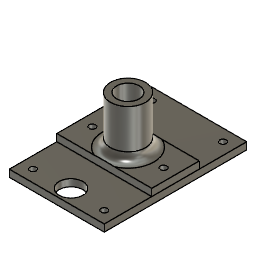
receiver_lens_15mm (Autodesk Fusion 360 design; units mm, degrees)
Autodesk Fusion 360 part; units mm, degrees
sketch "Sketch1" plane through (0, 0, 0) normal (0, 0, 1) x (1, 0, 0)
  circle A0 centre (20, 6) radius 5
  line L0 (0, 60) -> (0, 0)
  line L1 (40, 60) -> (0, 60)
  circle A1 centre (20, 30) radius 4.75
  line L2 (40, 0) -> (40, 60)
  circle A2 centre (35, 55) radius 1.35
  line L3 (0, 0) -> (40, 0)
  circle A3 centre (35, 5) radius 1.35
  circle A4 centre (20, 30) radius 6.25
  circle A5 centre (5, 5) radius 1.35
  circle A6 centre (5, 30) radius 1.35
  circle A7 centre (35, 30) radius 1.35
  circle A8 centre (5, 55) radius 1.35
  circle A9 centre (20, 30) radius 5.5
  dimension "d3" = 30
  dimension "d4" = 50
  dimension "d9" = 2.7
  dimension "d10" = 60
  dimension "d11" = 40
  dimension "d12" = 5
  dimension "d13" = 5
  dimension "d14" = 12.5
  dimension "d15" = 20
  dimension "d16" = 30
  dimension "d17" = 9.5
  dimension "d18" = 6
  dimension "d19" = 20
  dimension "d20" = 10
  dimension "d32" = 11
  constraint horizontal L3
  constraint vertical L2
  constraint horizontal L1
  constraint vertical L0
  constraint coincident L0.end L3.start
  constraint concentric A1 A4
  constraint concentric A4 A9
  measures "d9" diameter of A5
  measures "d10" distance of L2.start L1.start
  measures "d11" distance of L0.start L1.start
  measures "d12" distance of A5.centre L3
  measures "d13" distance of A5.centre L0
  measures "d14" diameter of A4
  measures "d15" distance of A1.centre L2
  measures "d16" distance of A1.centre L3
  measures "d17" diameter of A1
  measures "d18" distance of A0.centre L3
  measures "d19" distance of A0.centre L2
  measures "d20" diameter of A0
  measures "d32" diameter of A9
extrude "Extrude1" add sketch "Sketch1" along normal blind 3 contours L0 L1 L2 L3 makes body 1
extrude "Extrude2" add sketch "Sketch1" along normal blind 14 separate body contours A4 | A9 makes body 2
sketch "Sketch2" plane through (0, 0, 14) normal (0, 0, 1) x (-1, 0, 0)
  circle A0 centre (-20, -30) radius 4.75
  circle A1 centre (-20, -30) radius 6.25
  circle A2 centre (-20, -30) radius 5.5
  dimension "d33" = 11
  constraint concentric A0 A2
  measures "d33" diameter of A2
extrude "Extrude3" cut sketch "Sketch2" against normal blind 1 contours A2 bodies 2
sketch "Sketch3" plane through (0, 0, 3) normal (0, 0, 1) x (-1, 0, 0)
  circle A0 centre (-20, -30) radius 6.25
  circle A1 centre (-35, -5) radius 1.35
  circle A2 centre (-5, -55) radius 1.35
  circle A3 centre (-20, -6) radius 5
  circle A4 centre (-5, -30) radius 1.35
  circle A5 centre (-35, -30) radius 1.35
  circle A6 centre (-35, -55) radius 1.35
  circle A7 centre (-5, -5) radius 1.35
  line L0 (0, 0) -> (-40, 0)
  line L1 (-40, 0) -> (-40, -60)
  line L2 (-40, -60) -> (0, -60)
  line L3 (0, -60) -> (0, 0)
  line L4 (0, -40) -> (-40, -40)
  line L5 (-40, -40) -> (-40, -20)
  line L6 (-40, -20) -> (0, -20)
  line L7 (0, -20) -> (0, -40)
  line L8 (0, 0) -> (-40, 0)
  circle A8 centre (-20, -30) radius 6.75
  circle A9 centre (-20, -30) radius 7.35
  circle A10 centre (-35, -30) radius 1.35
  circle A11 centre (-5, -30) radius 1.35
  dimension "d36" = 20
  dimension "d37" = 20
  dimension "d38" = 14.7
  dimension "d39" = 13.5
  constraint horizontal L4
  constraint vertical L5
  constraint horizontal L6
  constraint vertical L7
  constraint coincident L1 L5.end
  constraint coincident L3 L4.start
  constraint concentric A0 A8
  constraint concentric A8 A9
  constraint concentric A5 A10
  constraint concentric A4 A11
  measures "d36" distance of L4.end L5.end
  measures "d37" distance of L6 L8
  measures "d38" diameter of A9
  measures "d39" diameter of A8
extrude "Extrude4" add sketch "Sketch3" along normal blind 3 contours L1 L3 L4 L5 L6 L7 bodies 1
extrude "Extrude5" add sketch "Sketch3" along normal blind 23 contours A9 bodies 1
sketch "Sketch4" plane through (0, 0, 26) normal (0, 0, 1) x (-1, 0, 0)
  circle A0 centre (-20, -30) radius 6.75
  circle A1 centre (-20, -30) radius 7.35
  circle A2 centre (-20, -30) radius 4.75
  dimension "d44" = 9.5
  constraint concentric A0 A2
  measures "d44" diameter of A2
extrude "Extrude6" add sketch "Sketch4" against normal blind 10.5 contours A0 bodies 1
fillet "Fillet2" radius 1.5 1 edges at (26.2932, 32.4409, 15.5) on bodies 1
split "Split1" by plane through (0, 0, 3) normal (0, 0, 1) bodies 1 makes body 3 at (12.6865, 30.7318, 19.3333)
combine "Combine1" operation add target body 2 tool bodies 1
fillet "Fillet3" radius 3.5 1 edges at (26.2932, 32.4409, 3) on bodies 3
fillet "Fillet4" radius 2 1 edges at (14.173, 27.7399, 3) on bodies 2
fillet "Fillet5" radius 3.5 1 edges at (26.8526, 27.3421, 6) on bodies 3
move_body "Move1" bodies 3 to x (1, 0, 0) y (0, 1, 0) z (0, 0, 1) at (0, 0, 10)
sketch "Sketch5" plane through (0, 0, 14) normal (0, 0, 1) x (-1, 0, 0)
  circle A0 centre (-20, -30) radius 5.5
  circle A1 centre (-20, -30) radius 6.25
  circle A2 centre (-20, -30) radius 6.25
  circle A3 centre (-20, -30) radius 5.5
  circle A4 centre (-20, -30) radius 4.75
  dimension "d59" = 12.5
  dimension "d60" = 11
  dimension "d61" = 9.5
  constraint concentric A0 A2
  constraint concentric A0 A3
  constraint concentric A0 A4
  measures "d59" diameter of A2
  measures "d60" diameter of A3
  measures "d61" diameter of A4
extrude "Extrude7" add sketch "Sketch5" along normal blind 10 separate body contours A1 A2 makes body 4
extrude "Extrude8" add sketch "Sketch5" along normal blind 9 contours A0 A3 bodies 2 4
ref_plane "WorkPlane1" through (20, 30, 14) normal (0, 0, -1) x (-1, 0, 0)
split "Split2" by plane through (20, 30, 14) normal (0, 0, -1) bodies 2 makes body 5 at (19.8817, 47.9803, 0)
sketch "Sketch6" plane through (0, 0, 3) normal (0, 0, 1) x (-1, 0, 0)
  line L0 (0, -60) -> (0, 0)
  line L1 (0, 0) -> (-40, 0)
  line L2 (-40, 0) -> (-40, -60)
  line L3 (-40, -60) -> (0, -60)
  circle A0 centre (-5, -5) radius 1.35
  circle A1 centre (-20, -6) radius 5
  circle A2 centre (-35, -5) radius 1.35
  circle A3 centre (-35, -55) radius 1.35
  circle A4 centre (-5, -55) radius 1.35
  circle A5 centre (-35, -30) radius 1.35
  circle A6 centre (-5, -30) radius 1.35
  circle A7 centre (-20, -30) radius 8.25
  line L4 (0, -36) -> (-10, -36)
  line L5 (-10, -36) -> (-10, -24)
  line L6 (-10, -24) -> (0, -24)
  line L7 (0, -24) -> (0, -36)
  circle A8 centre (-5, -30) radius 1.3
  dimension "d65" = 2.6
  dimension "d66" = 10
  dimension "d67" = 12
  dimension "d68" = 6
  constraint horizontal L4
  constraint vertical L5
  constraint horizontal L6
  constraint vertical L7
  constraint coincident L0 L4.start
  constraint concentric A6 A8
  measures "d65" diameter of A8
  measures "d66" distance of L4.start L4.end
  measures "d67" distance of L4.start L6.end
  measures "d68" distance of L4 A6.centre
extrude "Extrude9" add sketch "Sketch6" along normal blind 10 separate body contours L0 L4 L5 L6 L7 makes body 6
ref_plane "WorkPlane2" through (20, 0, 0) normal (1, 0, 0) x (0, 1, 0)
mirror "Mirror1" about plane through (20, 0, 0) normal (1, 0, 0) of bodies 6 makes body 7
sketch "Sketch7" plane through (0, 0, 14) normal (0, 0, -1) x (1, 0, 0)
  circle A0 centre (20, -30) radius 6.25
  circle A1 centre (20, -30) radius 4.75
  circle A2 centre (20, -30) radius 5.25
  dimension "d74" = 10.5
  constraint concentric A0 A2
  measures "d74" diameter of A2
extrude "Extrude10" add sketch "Sketch7" along normal blind 0.75 contours A2 bodies 2
move_body "Move2" bodies 3 to x (1, 0, 0) y (0, 1, 0) z (0, 0, 1) at (0, 0, -10)
hidden bodies 2 6 7
